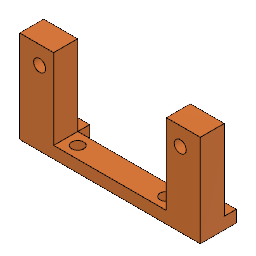
Fixateur pas a pas (Autodesk Fusion 360 design; units mm, degrees)
Autodesk Fusion 360 part; units mm, degrees
sketch "Sketch principal" plane through (0, 0, 0) normal (0, 0, 1) x (1, 0, 0)
  line L0 (45, 0) -> (45, 23)
  line L1 (45, 23) -> (36.5, 23)
  line L2 (36.5, 0) -> (45, 0)
  line L3 (36.5, 23) -> (36.5, 0)
  circle A0 centre (40, 18.5) radius 1.5
  line L4 (8.5, 23) -> (0, 23)
  line L5 (0, 0) -> (8.5, 0)
  line L6 (0, 23) -> (0, 0)
  line L7 (8.5, 0) -> (8.5, 23)
  circle A1 centre (5, 18.5) radius 1.5
  line L8 (8.5, 0) -> (36.5, 0)
  line L9 (36.5, 0) -> (36.5, 3)
  line L10 (36.5, 3) -> (8.5, 3)
  line L11 (8.5, 3) -> (8.5, 0)
  line L12 (8.5, 3) -> (0, 3)
  line L13 (0, 3) -> (0, 0)
  line L14 (0, 0) -> (8.5, 0)
  line L15 (8.5, 0) -> (8.5, 3)
  line L16 (36.5, 3) -> (45, 3)
  line L17 (45, 3) -> (45, 0)
  line L18 (45, 0) -> (36.5, 0)
  line L19 (36.5, 0) -> (36.5, 3)
  point P0 (36.5, 0)
  dimension "d15" = 23
  dimension "d16" = 8.5
  dimension "d17" = 3
  dimension "d18" = 4.5
  dimension "d20" = 23
  dimension "d21" = 8.5
  dimension "d22" = 3
  dimension "d23" = 4.5
  dimension "d24" = 3.5
  dimension "d25" = 28
  dimension "d26" = 3.5
  dimension "d28" = 3
  dimension "d29" = 28
  constraint horizontal L2
  constraint vertical L0
  constraint horizontal L1
  constraint vertical L3
  constraint coincident P0 L2.start
  constraint horizontal L5
  constraint vertical L7
  constraint horizontal L4
  constraint vertical L6
  constraint coincident L5.start L6.end
  constraint horizontal L8
  constraint vertical L9
  constraint horizontal L10
  constraint vertical L11
  constraint horizontal L12
  constraint vertical L13
  constraint horizontal L14
  constraint vertical L15
  constraint horizontal L16
  constraint vertical L17
  constraint horizontal L18
  constraint vertical L19
  measures "d15" distance of P0 L1.end
  measures "d16" distance of P0 L0.start
  measures "d17" diameter of A0
  measures "d18" distance of A0.centre L1
  measures "d20" distance of L5.start L4.end
  measures "d21" distance of L5.start L5.end
  measures "d22" diameter of A1
  measures "d23" distance of A1.centre L4
  measures "d24" distance of A1.centre L7
  measures "d25" distance of L3 L7
  measures "d26" distance of A0.centre L3
  measures "d28" distance of L5.end L10.end
  measures "d29" distance of L9.end L10.end
extrude "Extrude affichage" add sketch "Sketch principal" along normal blind 6
ref_plane "WorkPlane1" through (22.5, 13, 3) normal (1, 0, 0) x (0, 1, 0)
ref_plane "WorkPlane2" through (22.5, 11.5, 3) normal (0, 0, -1) x (-1, 0, 0)
sketch "Sketch4" plane through (0, 3, 0) normal (0, 1, 0) x (-1, 0, 0)
  line L0 (-36.5, 0) -> (-8.5, 0)
  line L1 (-8.5, 0) -> (-8.5, 6)
  line L2 (-8.5, 6) -> (-36.5, 6)
  line L3 (-36.5, 6) -> (-36.5, 0)
  circle A0 centre (-11.5, 3) radius 1.5
  line L4 (-22.5, 0) -> (-22.5, 6)
  circle A1 centre (-33.5, 3) radius 1.5
  dimension "d32" = 3
  dimension "d35" = 3
  constraint midpoint L0 L4.start
  constraint midpoint L2 L4.end
  constraint symmetric A0 L4 A1
  measures "d32" diameter of A0
  measures "d35" distance of L1 A0.centre
extrude "Extrude2" cut sketch "Sketch4" against normal blind 11 contours A0 | A1
extrude "Extrude3" add sketch "Sketch principal" against normal blind 3 contours L0 L2 L3 L9 L16 L17 L18 L19 | L5 L6 L7 L11 L12 L13 L14 L15
named bodies: "Fixateur U"
